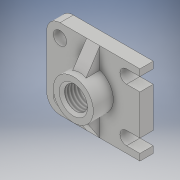
# Autodesk Inventor part: Основание
Saved by Autodesk Inventor 2019.3 (Build 233278000, 278)
## iProperties
Created: 2020-04-03
Part Number: Основание
Material: Типовые
Document SubType Name: Modeling
Designer: Admin
Density: 1 g/cm^3
Appearance: По умолчанию
Mass: 43.3813 g
Surface Area: 135.326 cm^2
Volume: 43.3813 cm^3
Author: Admin
Autodesk Inventor part; units mm, degrees
ref_plane "XY Plane" through (0, 0, 0) normal (0, 0, 1) x (1, 0, 0)
sketch "Эскиз1" plane through (0, 0, 0) normal (0, 0, 1) x (1, 0, 0)
  line L0 (70, 60) -> (10, 60)
  line L1 (0, 50) -> (0, 10)
  line L2 (10, 0) -> (70, 0)
  line L3 (70, 0) -> (70, 5)
  line L4 (70, 5) -> (60, 5)
  line L5 (70, 60) -> (70, 55)
  line L6 (70, 55) -> (60, 55)
  line L7 (60, 45) -> (70, 45)
  line L8 (70, 45) -> (70, 15)
  line L9 (70, 15) -> (60, 15)
  arc A0 (60, 55) -> (60, 45) centre (60, 50) ccw
  arc A1 (60, 15) -> (60, 5) centre (60, 10) ccw
  arc A2 (10, 60) -> (0, 50) centre (10, 50) ccw
  arc A3 (0, 10) -> (10, 0) centre (10, 10) ccw
  point P0 (0, 0)
  point P1 (0, 0)
  dimension "d0" = 5
  dimension "d1" = 5
  dimension "d2" = 10
  dimension "d3" = 10
  dimension "d4" = 40
  dimension "d5" = 60
  dimension "d6" = 70
  dimension "d7" = 10
  dimension "d8" = 10
  constraints: 20 end point, 8 point on circle, 6 horizontal, 6 vertical alignment, 4 centre point, 4 tangent, 4 vertical, 2 point on line, 1 coincident, 1 collinear
  measures "d0" radius of A0
  measures "d1" radius of A1
  measures "d2" distance between parallel lines of L7 L6
  measures "d3" radius of A2
  measures "d4" distance of A1.centre A0.centre
  measures "d5" distance between parallel lines of L2 L0
  measures "d6" distance between parallel lines of L8 L1
  measures "d7" distance of L5.end L6.end
  measures "d8" radius of A3
extrude "Выдавливание1" add sketch "Эскиз1" along normal blind 10
sketch "Эскиз2" plane through (0, 0, 10) normal (0, 0, 1) x (1, 0, 0)
  circle A0 centre (35, 30) radius 15
  line L0 (0, 50) -> (0, 10) projected
  line L1 (70, 55) -> (70, 60) projected
  point P0 (0, 0)
  point P1 (0, 30)
  dimension "d11" = 30
  dimension "d12" = 35
  constraints: 1 centre point, 1 horizontal alignment, 1 midpoint
  measures "d11" diameter of A0
  measures "d12" distance from line of L1 A0.centre
extrude "Выдавливание2" add sketch "Эскиз2" along normal blind 15
sketch "Эскиз3" plane through (0, 0, 10) normal (0, 0, 1) x (1, 0, 0)
  circle A0 centre (35, 30) radius 15 projected
  line L0 (70, 60) -> (10, 60) projected
  point P0 (0, 0)
  point P1 (10, 50)
  point P2 (10, 10)
  dimension "d15" = 40
  dimension "d16" = 25
  dimension "d17" = 10
  constraints: 1 vertical alignment
  measures "d15" distance of point (10, 10) point (10, 50)
  measures "d16" horizontal distance of A0.centre point (10, 50)
  measures "d17" distance from line of L0 point (10, 50)
hole "Отверстие1" at (10, 50, 10) at (10, 10, 10) direction (0, 0, -1) diameter 10 end through all
sketch "Эскиз4" plane through (35, 30, 25) normal (0, 0, 1) x (1, 0, 0)
  point P0 (-35, -30)
  point P1 (0, 0)
hole "Отверстие2" at (35, 30, 25) direction (0, 0, -1) diameter 17.3 end through all
chamfer "Фаска1" distance 2 angle 45 1 edges at (35, 38.65, 25)
ref_plane "РабПлоскость1" through (35, 0, 0) normal (1, 0, 0) x (0, 1, 0)
sketch "Эскиз5" plane through (35, 0, 0) normal (1, 0, 0) x (0, 1, 0)
  line L0 (15, 10) -> (15, 25) projected
  line L1 (15, 20) -> (0, 10)
  point P0 (0, 0)
  dimension "d36" = 5
  constraints: 2 end point, 1 coincident, 1 point on line
  measures "d36" distance of L0.end L1.start
ref_plane "РабПлоскость2" through (0, 30, 0) normal (0, 1, 0) x (-1, 0, 0)
extrude "Ребро жесткости2" add sketch "Эскиз5" along normal mid plane 10 rib yes fills toward (7.5277, 14.9584) open curves L1
mirror "Зеркальное отражение2" about plane through (0, 30, 0) normal (0, 1, 0) of "Ребро жесткости2"
